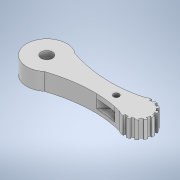
# Autodesk Inventor part: SPRINGGY_LEG
Saved by Autodesk Inventor 2020.3 (Build 243373000, 373)
## iProperties
Created: 2020-07-22
Part Number: SPRINGGY_LEG
Material: Generic
Document SubType Name: Modeling
Designer: aditk
Density: 1 g/cm^3
Appearance: Default
Author: aditk
Autodesk Inventor part; units mm, degrees
ref_plane "YZ Plane" through (0, 0, 0) normal (1, 0, 0) x (0, 1, 0)
ref_plane "XZ Plane" through (0, 0, 0) normal (0, 1, 0) x (-1, 0, 0)
ref_plane "XY Plane" through (0, 0, 0) normal (0, 0, 1) x (1, 0, 0)
sketch "Sketch1" plane through (0, 0, 0) normal (0, 1, 0) x (-1, 0, 0)
  arc A0 (-2.2387, -2.6904) -> (-2.2387, 2.6904) centre (0, 0) ccw
  arc A1 (-14.7206, 2.0922) -> (-14.7206, -2.0922) centre (-16.0891, 0) ccw
  spline S0 degree 2 poles (-14.7206, -2.0922) (-8.865, -0.5746) (-2.2387, -2.6904) knots 1.091642 1.091642 1.091642 1.869812 1.869812 1.869812
  spline S1 degree 2 poles (-14.7206, 2.0922) (-8.865, 0.5746) (-2.2387, 2.6904) knots 1.091642 1.091642 1.091642 1.869812 1.869812 1.869812
  line L0 (-14.7206, 2.0922) -> (-8.865, 0.5746) construction
  line L1 (-14.7206, -2.0922) -> (-8.865, -0.5746) construction
  line L2 (-8.865, -0.5746) -> (-2.2387, -2.6904) construction
  line L3 (-8.865, 0.5746) -> (-2.2387, 2.6904) construction
  circle A2 centre (-12.1383, 0) radius 0.5
  point P0 (-4.1001, 12.1141)
  dimension "d0" = 7
  dimension "d1" = 5
  dimension "d2" = 1
  constraints: 4 point on circle, 3 centre point, 2 coincident, 6 other
  measures "d0" diameter of A0
  measures "d1" diameter of A1
  measures "d2" diameter of A2
extrude "Extrusion1" add sketch "Sketch1" along normal blind 3
sketch "Sketch2" plane through (0, 3, 0) normal (0, 1, 0) x (1, 0, 0)
  circle A0 centre (0, 0) radius 1
  line L0 (16.3636, -2.5462) -> (15.8145, -2.5462)
  arc A1 (14.7206, -2.0922) -> (14.7206, 2.0922) centre (16.0891, 0) ccw projected
  line L1 (15.8145, -2.5462) -> (15.8145, -2.14)
  line L2 (16.3636, -2.14) -> (16.3636, -2.5462)
  arc A2 (15.8145, -2.14) -> (16.3636, -2.14) centre (16.0891, 0) ccw
  arc A3 (16.7702, -2.0472) -> (17.2649, -1.8089) centre (16.0891, 0) ccw
  line L3 (16.9465, -2.4131) -> (16.7702, -2.0472)
  line L4 (17.2649, -1.8089) -> (17.4411, -2.1749)
  line L5 (17.4411, -2.1749) -> (16.9465, -2.4131)
  arc A4 (17.591, -1.5489) -> (17.9333, -1.1196) centre (16.0891, 0) ccw
  line L6 (17.9086, -1.8021) -> (17.591, -1.5489)
  line L7 (17.9333, -1.1196) -> (18.2509, -1.3729)
  line L8 (18.2509, -1.3729) -> (17.9086, -1.8021)
  arc A5 (18.1143, -0.7438) -> (18.2365, -0.2085) centre (16.0891, 0) ccw
  line L9 (18.5103, -0.8342) -> (18.1143, -0.7438)
  line L10 (18.2365, -0.2085) -> (18.6325, -0.2989)
  line L11 (18.6325, -0.2989) -> (18.5103, -0.8342)
  arc A6 (18.2365, 0.2085) -> (18.1143, 0.7438) centre (16.0891, 0) ccw
  line L12 (18.6325, 0.2989) -> (18.2365, 0.2085)
  line L13 (18.1143, 0.7438) -> (18.5103, 0.8342)
  line L14 (18.5103, 0.8342) -> (18.6325, 0.2989)
  arc A7 (17.9333, 1.1196) -> (17.591, 1.5489) centre (16.0891, 0) ccw
  line L15 (18.2509, 1.3729) -> (17.9333, 1.1196)
  line L16 (17.591, 1.5489) -> (17.9086, 1.8021)
  line L17 (17.9086, 1.8021) -> (18.2509, 1.3729)
  arc A8 (17.2649, 1.8089) -> (16.7702, 2.0472) centre (16.0891, 0) ccw
  line L18 (17.4411, 2.1749) -> (17.2649, 1.8089)
  line L19 (16.7702, 2.0472) -> (16.9465, 2.4131)
  line L20 (16.9465, 2.4131) -> (17.4411, 2.1749)
  arc A9 (16.3636, 2.14) -> (15.8145, 2.14) centre (16.0891, 0) ccw
  line L21 (16.3636, 2.5462) -> (16.3636, 2.14)
  line L22 (15.8145, 2.14) -> (15.8145, 2.5462)
  line L23 (15.8145, 2.5462) -> (16.3636, 2.5462)
  dimension "d5" = 2
  dimension "d8" = 180
  constraints: 48 end point, 16 point on circle, 9 centre point, 2 coincident, 1 parallel, 1 perpendicular, 1 vertical, 63 other
  measures "d5" diameter of A0
extrude "Extrusion2" cut sketch "Sketch2" against normal up to next
sketch "Sketch3" plane through (0, 3, 0) normal (0, 1, 0) x (1, 0, 0)
  circle A0 centre (12.1383, 0) radius 0.5 projected
  line L0 (12.1383, 0) -> (12.1383, -1.6187)
  line L1 (12.1383, 0) -> (14.0705, 0) construction
  line L2 (12.1383, 0) -> (10.2334, -1.9049)
  line L3 (12.1383, 0) -> (14.8323, 0) construction
  line L4 (11.6383, 0) -> (10.1304, -1.5079)
  line L5 (12.6383, 0) -> (14.1463, -1.5079)
  line L6 (14.1463, -1.5079) -> (14.0705, -1.5837)
  line L7 (14.0705, -1.5837) -> (13.7493, -1.9049)
  line L8 (13.7493, -1.9049) -> (10.1304, -1.5079)
  point P0 (0, 0)
  dimension "d13" = 135
  constraints: 18 end point, 2 horizontal, 2 symmetric about line, 1 equal length, 1 point on line, 1 vertical, 2 other
  measures "d13" angle of L2 L3
extrude "Extrusion3" cut sketch "Sketch3" against normal blind 2.3 contours L5 L6 L7 L8 L2 A0 | A0 L2 L8 L4
sketch "Sketch4" plane through (0, 3, 0) normal (0, 1, 0) x (1, 0, 0)
  spline S0 degree 7 poles (13.7811, -1.8731) (13.7774, -1.8723) (13.7736, -1.8716) (13.7699, -1.8708) (13.7662, -1.87) (13.7625, -1.8693) (13.7588, -1.8685) (13.7297, -1.8625) (13.7043, -1.8573) (13.6789, -1.8522) (13.6535, -1.8471) (13.6281, -1.842) (13.6027, -1.837) (13.097, -1.7376) (12.6139, -1.6572) (12.1285, -1.5908) (11.6414, -1.5384) (11.1531, -1.4999) (10.6639, -1.4751) (10.1745, -1.4638) knots 0 0 0 0 0 0 0 0 0.007311 0.007311 0.007311 0.007311 0.007311 0.007311 0.057193 0.057193 0.057193 0.057193 0.057193 0.057193 1 1 1 1 1 1 1 1 projected
  line L0 (14.1463, -1.5079) -> (13.7811, -1.8731) projected
  line L1 (12.6383, 0) -> (14.1463, -1.5079) projected
  arc A0 (11.6383, 0) -> (12.6383, 0) centre (12.1383, 0) ccw projected
  line L2 (10.1745, -1.4638) -> (11.6383, 0) projected
  point P0 (0, 0)
  constraints: 1 other
extrude "Extrusion4" add sketch "Sketch4" against normal blind 0.8
body "Solid1"
